Autodesk Inventor part; units mm, degrees
(part 2 of 3)
  line L469 (15.7875, 18.7015) -> (16.0329, 18.7015) construction
  spline S155 degree 3 poles (16.0329, 18.7015) (16.2784, 18.7015) (16.4775, 18.9006) (16.4775, 19.1461) knots 0 0 0 0 1 1 1 1
  line L470 (16.0329, 18.7015) -> (16.2784, 18.7015) construction
  line L471 (16.2784, 18.7015) -> (16.4775, 18.9006) construction
  line L472 (16.4775, 18.9006) -> (16.4775, 19.1461) construction
  spline S156 degree 3 poles (11.3975, 19.1461) (11.3975, 19.3915) (11.1984, 19.5905) (10.9529, 19.5905) knots 0 0 0 0 1 1 1 1
  line L473 (11.3975, 19.1461) -> (11.3975, 19.3915) construction
  line L474 (11.3975, 19.3915) -> (11.1984, 19.5905) construction
  line L475 (11.1984, 19.5905) -> (10.9529, 19.5905) construction
  spline S157 degree 3 poles (10.9529, 19.5905) (10.7075, 19.5905) (10.5085, 19.3915) (10.5085, 19.1461) knots 0 0 0 0 1 1 1 1
  line L476 (10.9529, 19.5905) -> (10.7075, 19.5905) construction
  line L477 (10.7075, 19.5905) -> (10.5085, 19.3915) construction
  line L478 (10.5085, 19.3915) -> (10.5085, 19.1461) construction
  spline S158 degree 3 poles (10.5085, 19.1461) (10.5085, 18.9006) (10.7075, 18.7015) (10.9529, 18.7015) knots 0 0 0 0 1 1 1 1
  line L479 (10.5085, 19.1461) -> (10.5085, 18.9006) construction
  line L480 (10.5085, 18.9006) -> (10.7075, 18.7015) construction
  line L481 (10.7075, 18.7015) -> (10.9529, 18.7015) construction
  spline S159 degree 3 poles (10.9529, 18.7015) (11.1984, 18.7015) (11.3975, 18.9006) (11.3975, 19.1461) knots 0 0 0 0 1 1 1 1
  line L482 (10.9529, 18.7015) -> (11.1984, 18.7015) construction
  line L483 (11.1984, 18.7015) -> (11.3975, 18.9006) construction
  line L484 (11.3975, 18.9006) -> (11.3975, 19.1461) construction
  spline S160 degree 3 poles (8.8575, 19.1461) (8.8575, 19.3915) (8.6584, 19.5905) (8.4129, 19.5905) knots 0 0 0 0 1 1 1 1
  line L485 (8.8575, 19.1461) -> (8.8575, 19.3915) construction
  line L486 (8.8575, 19.3915) -> (8.6584, 19.5905) construction
  line L487 (8.6584, 19.5905) -> (8.4129, 19.5905) construction
  spline S161 degree 3 poles (8.4129, 19.5905) (8.1675, 19.5905) (7.9685, 19.3915) (7.9685, 19.1461) knots 0 0 0 0 1 1 1 1
  line L488 (8.4129, 19.5905) -> (8.1675, 19.5905) construction
  line L489 (8.1675, 19.5905) -> (7.9685, 19.3915) construction
  line L490 (7.9685, 19.3915) -> (7.9685, 19.1461) construction
  spline S162 degree 3 poles (7.9685, 19.1461) (7.9685, 18.9006) (8.1675, 18.7015) (8.4129, 18.7015) knots 0 0 0 0 1 1 1 1
  line L491 (7.9685, 19.1461) -> (7.9685, 18.9006) construction
  line L492 (7.9685, 18.9006) -> (8.1675, 18.7015) construction
  line L493 (8.1675, 18.7015) -> (8.4129, 18.7015) construction
  spline S163 degree 3 poles (8.4129, 18.7015) (8.6584, 18.7015) (8.8575, 18.9006) (8.8575, 19.1461) knots 0 0 0 0 1 1 1 1
  line L494 (8.4129, 18.7015) -> (8.6584, 18.7015) construction
  line L495 (8.6584, 18.7015) -> (8.8575, 18.9006) construction
  line L496 (8.8575, 18.9006) -> (8.8575, 19.1461) construction
  spline S164 degree 3 poles (6.3175, 19.1461) (6.3175, 19.3915) (6.1184, 19.5905) (5.8729, 19.5905) knots 0 0 0 0 1 1 1 1
  line L497 (6.3175, 19.1461) -> (6.3175, 19.3915) construction
  line L498 (6.3175, 19.3915) -> (6.1184, 19.5905) construction
  line L499 (6.1184, 19.5905) -> (5.8729, 19.5905) construction
  spline S165 degree 3 poles (5.8729, 19.5905) (5.6275, 19.5905) (5.4285, 19.3915) (5.4285, 19.1461) knots 0 0 0 0 1 1 1 1
  line L500 (5.8729, 19.5905) -> (5.6275, 19.5905) construction
  line L501 (5.6275, 19.5905) -> (5.4285, 19.3915) construction
  line L502 (5.4285, 19.3915) -> (5.4285, 19.1461) construction
  spline S166 degree 3 poles (5.4285, 19.1461) (5.4285, 18.9006) (5.6275, 18.7015) (5.8729, 18.7015) knots 0 0 0 0 1 1 1 1
  line L503 (5.4285, 19.1461) -> (5.4285, 18.9006) construction
  line L504 (5.4285, 18.9006) -> (5.6275, 18.7015) construction
  line L505 (5.6275, 18.7015) -> (5.8729, 18.7015) construction
  spline S167 degree 3 poles (5.8729, 18.7015) (6.1184, 18.7015) (6.3175, 18.9006) (6.3175, 19.1461) knots 0 0 0 0 1 1 1 1
  line L506 (5.8729, 18.7015) -> (6.1184, 18.7015) construction
  line L507 (6.1184, 18.7015) -> (6.3175, 18.9006) construction
  line L508 (6.3175, 18.9006) -> (6.3175, 19.1461) construction
  spline S168 degree 3 poles (6.3175, 15.3361) (6.3175, 15.5815) (6.1184, 15.7805) (5.8729, 15.7805) knots 0 0 0 0 1 1 1 1
  line L509 (6.3175, 15.3361) -> (6.3175, 15.5815) construction
  line L510 (6.3175, 15.5815) -> (6.1184, 15.7805) construction
  line L511 (6.1184, 15.7805) -> (5.8729, 15.7805) construction
  spline S169 degree 3 poles (5.8729, 15.7805) (5.6275, 15.7805) (5.4285, 15.5815) (5.4285, 15.3361) knots 0 0 0 0 1 1 1 1
  line L512 (5.8729, 15.7805) -> (5.6275, 15.7805) construction
  line L513 (5.6275, 15.7805) -> (5.4285, 15.5815) construction
  line L514 (5.4285, 15.5815) -> (5.4285, 15.3361) construction
  spline S170 degree 3 poles (5.4285, 15.3361) (5.4285, 15.0906) (5.6275, 14.8915) (5.8729, 14.8915) knots 0 0 0 0 1 1 1 1
  line L515 (5.4285, 15.3361) -> (5.4285, 15.0906) construction
  line L516 (5.4285, 15.0906) -> (5.6275, 14.8915) construction
  line L517 (5.6275, 14.8915) -> (5.8729, 14.8915) construction
  spline S171 degree 3 poles (5.8729, 14.8915) (6.1184, 14.8915) (6.3175, 15.0906) (6.3175, 15.3361) knots 0 0 0 0 1 1 1 1
  line L518 (5.8729, 14.8915) -> (6.1184, 14.8915) construction
  line L519 (6.1184, 14.8915) -> (6.3175, 15.0906) construction
  line L520 (6.3175, 15.0906) -> (6.3175, 15.3361) construction
  spline S172 degree 3 poles (8.8575, 15.3361) (8.8575, 15.5815) (8.6584, 15.7805) (8.4129, 15.7805) knots 0 0 0 0 1 1 1 1
  line L521 (8.8575, 15.3361) -> (8.8575, 15.5815) construction
  line L522 (8.8575, 15.5815) -> (8.6584, 15.7805) construction
  line L523 (8.6584, 15.7805) -> (8.4129, 15.7805) construction
  spline S173 degree 3 poles (8.4129, 15.7805) (8.1675, 15.7805) (7.9685, 15.5815) (7.9685, 15.3361) knots 0 0 0 0 1 1 1 1
  line L524 (8.4129, 15.7805) -> (8.1675, 15.7805) construction
  line L525 (8.1675, 15.7805) -> (7.9685, 15.5815) construction
  line L526 (7.9685, 15.5815) -> (7.9685, 15.3361) construction
  spline S174 degree 3 poles (7.9685, 15.3361) (7.9685, 15.0906) (8.1675, 14.8915) (8.4129, 14.8915) knots 0 0 0 0 1 1 1 1
  line L527 (7.9685, 15.3361) -> (7.9685, 15.0906) construction
  line L528 (7.9685, 15.0906) -> (8.1675, 14.8915) construction
  line L529 (8.1675, 14.8915) -> (8.4129, 14.8915) construction
  spline S175 degree 3 poles (8.4129, 14.8915) (8.6584, 14.8915) (8.8575, 15.0906) (8.8575, 15.3361) knots 0 0 0 0 1 1 1 1
  line L530 (8.4129, 14.8915) -> (8.6584, 14.8915) construction
  line L531 (8.6584, 14.8915) -> (8.8575, 15.0906) construction
  line L532 (8.8575, 15.0906) -> (8.8575, 15.3361) construction
  spline S176 degree 3 poles (19.0175, 19.1461) (19.0175, 19.3915) (18.8184, 19.5905) (18.5729, 19.5905) knots 0 0 0 0 1 1 1 1
  line L533 (19.0175, 19.1461) -> (19.0175, 19.3915) construction
  line L534 (19.0175, 19.3915) -> (18.8184, 19.5905) construction
  line L535 (18.8184, 19.5905) -> (18.5729, 19.5905) construction
  spline S177 degree 3 poles (18.5729, 19.5905) (18.3275, 19.5905) (18.1285, 19.3915) (18.1285, 19.1461) knots 0 0 0 0 1 1 1 1
  line L536 (18.5729, 19.5905) -> (18.3275, 19.5905) construction
  line L537 (18.3275, 19.5905) -> (18.1285, 19.3915) construction
  line L538 (18.1285, 19.3915) -> (18.1285, 19.1461) construction
  spline S178 degree 3 poles (18.1285, 19.1461) (18.1285, 18.9006) (18.3275, 18.7015) (18.5729, 18.7015) knots 0 0 0 0 1 1 1 1
  line L539 (18.1285, 19.1461) -> (18.1285, 18.9006) construction
  line L540 (18.1285, 18.9006) -> (18.3275, 18.7015) construction
  line L541 (18.3275, 18.7015) -> (18.5729, 18.7015) construction
  spline S179 degree 3 poles (18.5729, 18.7015) (18.8184, 18.7015) (19.0175, 18.9006) (19.0175, 19.1461) knots 0 0 0 0 1 1 1 1
  line L542 (18.5729, 18.7015) -> (18.8184, 18.7015) construction
  line L543 (18.8184, 18.7015) -> (19.0175, 18.9006) construction
  line L544 (19.0175, 18.9006) -> (19.0175, 19.1461) construction
  spline S180 degree 3 poles (21.5575, 19.1461) (21.5575, 19.3915) (21.3584, 19.5905) (21.1129, 19.5905) knots 0 0 0 0 1 1 1 1
  line L545 (21.5575, 19.1461) -> (21.5575, 19.3915) construction
  line L546 (21.5575, 19.3915) -> (21.3584, 19.5905) construction
  line L547 (21.3584, 19.5905) -> (21.1129, 19.5905) construction
  spline S181 degree 3 poles (21.1129, 19.5905) (20.8675, 19.5905) (20.6685, 19.3915) (20.6685, 19.1461) knots 0 0 0 0 1 1 1 1
  line L548 (21.1129, 19.5905) -> (20.8675, 19.5905) construction
  line L549 (20.8675, 19.5905) -> (20.6685, 19.3915) construction
  line L550 (20.6685, 19.3915) -> (20.6685, 19.1461) construction
  spline S182 degree 3 poles (20.6685, 19.1461) (20.6685, 18.9006) (20.8675, 18.7015) (21.1129, 18.7015) knots 0 0 0 0 1 1 1 1
  line L551 (20.6685, 19.1461) -> (20.6685, 18.9006) construction
  line L552 (20.6685, 18.9006) -> (20.8675, 18.7015) construction
  line L553 (20.8675, 18.7015) -> (21.1129, 18.7015) construction
  spline S183 degree 3 poles (21.1129, 18.7015) (21.3584, 18.7015) (21.5575, 18.9006) (21.5575, 19.1461) knots 0 0 0 0 1 1 1 1
  line L554 (21.1129, 18.7015) -> (21.3584, 18.7015) construction
  line L555 (21.3584, 18.7015) -> (21.5575, 18.9006) construction
  line L556 (21.5575, 18.9006) -> (21.5575, 19.1461) construction
  spline S184 degree 3 poles (24.0975, 19.1461) (24.0975, 19.3915) (23.8984, 19.5905) (23.6529, 19.5905) knots 0 0 0 0 1 1 1 1
  line L557 (24.0975, 19.1461) -> (24.0975, 19.3915) construction
  line L558 (24.0975, 19.3915) -> (23.8984, 19.5905) construction
  line L559 (23.8984, 19.5905) -> (23.6529, 19.5905) construction
  spline S185 degree 3 poles (23.6529, 19.5905) (23.4075, 19.5905) (23.2085, 19.3915) (23.2085, 19.1461) knots 0 0 0 0 1 1 1 1
  line L560 (23.6529, 19.5905) -> (23.4075, 19.5905) construction
  line L561 (23.4075, 19.5905) -> (23.2085, 19.3915) construction
  line L562 (23.2085, 19.3915) -> (23.2085, 19.1461) construction
  spline S186 degree 3 poles (23.2085, 19.1461) (23.2085, 18.9006) (23.4075, 18.7015) (23.6529, 18.7015) knots 0 0 0 0 1 1 1 1
  line L563 (23.2085, 19.1461) -> (23.2085, 18.9006) construction
  line L564 (23.2085, 18.9006) -> (23.4075, 18.7015) construction
  line L565 (23.4075, 18.7015) -> (23.6529, 18.7015) construction
  spline S187 degree 3 poles (23.6529, 18.7015) (23.8984, 18.7015) (24.0975, 18.9006) (24.0975, 19.1461) knots 0 0 0 0 1 1 1 1
  line L566 (23.6529, 18.7015) -> (23.8984, 18.7015) construction
  line L567 (23.8984, 18.7015) -> (24.0975, 18.9006) construction
  line L568 (24.0975, 18.9006) -> (24.0975, 19.1461) construction
  spline S188 degree 3 poles (11.3975, 15.3361) (11.3975, 15.5815) (11.1984, 15.7805) (10.9529, 15.7805) knots 0 0 0 0 1 1 1 1
  line L569 (11.3975, 15.3361) -> (11.3975, 15.5815) construction
  line L570 (11.3975, 15.5815) -> (11.1984, 15.7805) construction
  line L571 (11.1984, 15.7805) -> (10.9529, 15.7805) construction
  spline S189 degree 3 poles (10.9529, 15.7805) (10.7075, 15.7805) (10.5085, 15.5815) (10.5085, 15.3361) knots 0 0 0 0 1 1 1 1
  line L572 (10.9529, 15.7805) -> (10.7075, 15.7805) construction
  line L573 (10.7075, 15.7805) -> (10.5085, 15.5815) construction
  line L574 (10.5085, 15.5815) -> (10.5085, 15.3361) construction
  spline S190 degree 3 poles (10.5085, 15.3361) (10.5085, 15.0906) (10.7075, 14.8915) (10.9529, 14.8915) knots 0 0 0 0 1 1 1 1
  line L575 (10.5085, 15.3361) -> (10.5085, 15.0906) construction
  line L576 (10.5085, 15.0906) -> (10.7075, 14.8915) construction
  line L577 (10.7075, 14.8915) -> (10.9529, 14.8915) construction
  spline S191 degree 3 poles (10.9529, 14.8915) (11.1984, 14.8915) (11.3975, 15.0906) (11.3975, 15.3361) knots 0 0 0 0 1 1 1 1
  line L578 (10.9529, 14.8915) -> (11.1984, 14.8915) construction
  line L579 (11.1984, 14.8915) -> (11.3975, 15.0906) construction
  line L580 (11.3975, 15.0906) -> (11.3975, 15.3361) construction
  spline S192 degree 3 poles (13.9375, 15.3361) (13.9375, 15.5815) (13.7384, 15.7805) (13.4929, 15.7805) knots 0 0 0 0 1 1 1 1
  line L581 (13.9375, 15.3361) -> (13.9375, 15.5815) construction
  line L582 (13.9375, 15.5815) -> (13.7384, 15.7805) construction
  line L583 (13.7384, 15.7805) -> (13.4929, 15.7805) construction
  spline S193 degree 3 poles (13.4929, 15.7805) (13.2475, 15.7805) (13.0485, 15.5815) (13.0485, 15.3361) knots 0 0 0 0 1 1 1 1
  line L584 (13.4929, 15.7805) -> (13.2475, 15.7805) construction
  line L585 (13.2475, 15.7805) -> (13.0485, 15.5815) construction
  line L586 (13.0485, 15.5815) -> (13.0485, 15.3361) construction
  spline S194 degree 3 poles (13.0485, 15.3361) (13.0485, 15.0906) (13.2475, 14.8915) (13.4929, 14.8915) knots 0 0 0 0 1 1 1 1
  line L587 (13.0485, 15.3361) -> (13.0485, 15.0906) construction
  line L588 (13.0485, 15.0906) -> (13.2475, 14.8915) construction
  line L589 (13.2475, 14.8915) -> (13.4929, 14.8915) construction
  spline S195 degree 3 poles (13.4929, 14.8915) (13.7384, 14.8915) (13.9375, 15.0906) (13.9375, 15.3361) knots 0 0 0 0 1 1 1 1
  line L590 (13.4929, 14.8915) -> (13.7384, 14.8915) construction
  line L591 (13.7384, 14.8915) -> (13.9375, 15.0906) construction
  line L592 (13.9375, 15.0906) -> (13.9375, 15.3361) construction
  spline S196 degree 3 poles (16.4775, 15.3361) (16.4775, 15.5815) (16.2784, 15.7805) (16.0329, 15.7805) knots 0 0 0 0 1 1 1 1
  line L593 (16.4775, 15.3361) -> (16.4775, 15.5815) construction
  line L594 (16.4775, 15.5815) -> (16.2784, 15.7805) construction
  line L595 (16.2784, 15.7805) -> (16.0329, 15.7805) construction
  spline S197 degree 3 poles (16.0329, 15.7805) (15.7875, 15.7805) (15.5885, 15.5815) (15.5885, 15.3361) knots 0 0 0 0 1 1 1 1
  line L596 (16.0329, 15.7805) -> (15.7875, 15.7805) construction
  line L597 (15.7875, 15.7805) -> (15.5885, 15.5815) construction
  line L598 (15.5885, 15.5815) -> (15.5885, 15.3361) construction
  spline S198 degree 3 poles (15.5885, 15.3361) (15.5885, 15.0906) (15.7875, 14.8915) (16.0329, 14.8915) knots 0 0 0 0 1 1 1 1
  line L599 (15.5885, 15.3361) -> (15.5885, 15.0906) construction
  line L600 (15.5885, 15.0906) -> (15.7875, 14.8915) construction
  line L601 (15.7875, 14.8915) -> (16.0329, 14.8915) construction
  spline S199 degree 3 poles (16.0329, 14.8915) (16.2784, 14.8915) (16.4775, 15.0906) (16.4775, 15.3361) knots 0 0 0 0 1 1 1 1
  line L602 (16.0329, 14.8915) -> (16.2784, 14.8915) construction
  line L603 (16.2784, 14.8915) -> (16.4775, 15.0906) construction
  line L604 (16.4775, 15.0906) -> (16.4775, 15.3361) construction
  spline S200 degree 3 poles (19.0175, 15.3361) (19.0175, 15.5815) (18.8184, 15.7805) (18.5729, 15.7805) knots 0 0 0 0 1 1 1 1
  line L605 (19.0175, 15.3361) -> (19.0175, 15.5815) construction
  line L606 (19.0175, 15.5815) -> (18.8184, 15.7805) construction
  line L607 (18.8184, 15.7805) -> (18.5729, 15.7805) construction
  spline S201 degree 3 poles (18.5729, 15.7805) (18.3275, 15.7805) (18.1285, 15.5815) (18.1285, 15.3361) knots 0 0 0 0 1 1 1 1
  line L608 (18.5729, 15.7805) -> (18.3275, 15.7805) construction
  line L609 (18.3275, 15.7805) -> (18.1285, 15.5815) construction
  line L610 (18.1285, 15.5815) -> (18.1285, 15.3361) construction
  spline S202 degree 3 poles (18.1285, 15.3361) (18.1285, 15.0906) (18.3275, 14.8915) (18.5729, 14.8915) knots 0 0 0 0 1 1 1 1
  line L611 (18.1285, 15.3361) -> (18.1285, 15.0906) construction
  line L612 (18.1285, 15.0906) -> (18.3275, 14.8915) construction
  line L613 (18.3275, 14.8915) -> (18.5729, 14.8915) construction
  spline S203 degree 3 poles (18.5729, 14.8915) (18.8184, 14.8915) (19.0175, 15.0906) (19.0175, 15.3361) knots 0 0 0 0 1 1 1 1
  line L614 (18.5729, 14.8915) -> (18.8184, 14.8915) construction
  line L615 (18.8184, 14.8915) -> (19.0175, 15.0906) construction
  line L616 (19.0175, 15.0906) -> (19.0175, 15.3361) construction
  spline S204 degree 3 poles (21.5575, 15.3361) (21.5575, 15.5815) (21.3584, 15.7805) (21.1129, 15.7805) knots 0 0 0 0 1 1 1 1
  line L617 (21.5575, 15.3361) -> (21.5575, 15.5815) construction
  line L618 (21.5575, 15.5815) -> (21.3584, 15.7805) construction
  line L619 (21.3584, 15.7805) -> (21.1129, 15.7805) construction
  spline S205 degree 3 poles (21.1129, 15.7805) (20.8675, 15.7805) (20.6685, 15.5815) (20.6685, 15.3361) knots 0 0 0 0 1 1 1 1
  line L620 (21.1129, 15.7805) -> (20.8675, 15.7805) construction
  line L621 (20.8675, 15.7805) -> (20.6685, 15.5815) construction
  line L622 (20.6685, 15.5815) -> (20.6685, 15.3361) construction
  spline S206 degree 3 poles (20.6685, 15.3361) (20.6685, 15.0906) (20.8675, 14.8915) (21.1129, 14.8915) knots 0 0 0 0 1 1 1 1
  line L623 (20.6685, 15.3361) -> (20.6685, 15.0906) construction
  line L624 (20.6685, 15.0906) -> (20.8675, 14.8915) construction
  line L625 (20.8675, 14.8915) -> (21.1129, 14.8915) construction
  spline S207 degree 3 poles (21.1129, 14.8915) (21.3584, 14.8915) (21.5575, 15.0906) (21.5575, 15.3361) knots 0 0 0 0 1 1 1 1
  line L626 (21.1129, 14.8915) -> (21.3584, 14.8915) construction
  line L627 (21.3584, 14.8915) -> (21.5575, 15.0906) construction
  line L628 (21.5575, 15.0906) -> (21.5575, 15.3361) construction
  spline S208 degree 3 poles (24.0975, 15.3361) (24.0975, 15.5815) (23.8984, 15.7805) (23.6529, 15.7805) knots 0 0 0 0 1 1 1 1
  line L629 (24.0975, 15.3361) -> (24.0975, 15.5815) construction
  line L630 (24.0975, 15.5815) -> (23.8984, 15.7805) construction
  line L631 (23.8984, 15.7805) -> (23.6529, 15.7805) construction
  spline S209 degree 3 poles (23.6529, 15.7805) (23.4075, 15.7805) (23.2085, 15.5815) (23.2085, 15.3361) knots 0 0 0 0 1 1 1 1
  line L632 (23.6529, 15.7805) -> (23.4075, 15.7805) construction
  line L633 (23.4075, 15.7805) -> (23.2085, 15.5815) construction
  line L634 (23.2085, 15.5815) -> (23.2085, 15.3361) construction
  spline S210 degree 3 poles (23.2085, 15.3361) (23.2085, 15.0906) (23.4075, 14.8915) (23.6529, 14.8915) knots 0 0 0 0 1 1 1 1
  line L635 (23.2085, 15.3361) -> (23.2085, 15.0906) construction
  line L636 (23.2085, 15.0906) -> (23.4075, 14.8915) construction
  line L637 (23.4075, 14.8915) -> (23.6529, 14.8915) construction
  spline S211 degree 3 poles (23.6529, 14.8915) (23.8984, 14.8915) (24.0975, 15.0906) (24.0975, 15.3361) knots 0 0 0 0 1 1 1 1
  line L638 (23.6529, 14.8915) -> (23.8984, 14.8915) construction
  line L639 (23.8984, 14.8915) -> (24.0975, 15.0906) construction
  line L640 (24.0975, 15.0906) -> (24.0975, 15.3361) construction
  spline S212 degree 3 poles (13.9375, 29.3061) (13.9375, 29.5515) (13.7384, 29.7505) (13.4929, 29.7505) knots 0 0 0 0 1 1 1 1
  line L641 (13.9375, 29.3061) -> (13.9375, 29.5515) construction
  line L642 (13.9375, 29.5515) -> (13.7384, 29.7505) construction
  line L643 (13.7384, 29.7505) -> (13.4929, 29.7505) construction
  spline S213 degree 3 poles (13.4929, 29.7505) (13.2475, 29.7505) (13.0485, 29.5515) (13.0485, 29.3061) knots 0 0 0 0 1 1 1 1
  line L644 (13.4929, 29.7505) -> (13.2475, 29.7505) construction
  line L645 (13.2475, 29.7505) -> (13.0485, 29.5515) construction
  line L646 (13.0485, 29.5515) -> (13.0485, 29.3061) construction
  spline S214 degree 3 poles (13.0485, 29.3061) (13.0485, 29.0606) (13.2475, 28.8615) (13.4929, 28.8615) knots 0 0 0 0 1 1 1 1
  line L647 (13.0485, 29.3061) -> (13.0485, 29.0606) construction
  line L648 (13.0485, 29.0606) -> (13.2475, 28.8615) construction
  line L649 (13.2475, 28.8615) -> (13.4929, 28.8615) construction
  spline S215 degree 3 poles (13.4929, 28.8615) (13.7384, 28.8615) (13.9375, 29.0606) (13.9375, 29.3061) knots 0 0 0 0 1 1 1 1
  line L650 (13.4929, 28.8615) -> (13.7384, 28.8615) construction
  line L651 (13.7384, 28.8615) -> (13.9375, 29.0606) construction
  line L652 (13.9375, 29.0606) -> (13.9375, 29.3061) construction
  spline S216 degree 3 poles (16.4775, 29.3061) (16.4775, 29.5515) (16.2784, 29.7505) (16.0329, 29.7505) knots 0 0 0 0 1 1 1 1
  line L653 (16.4775, 29.3061) -> (16.4775, 29.5515) construction
  line L654 (16.4775, 29.5515) -> (16.2784, 29.7505) construction
  line L655 (16.2784, 29.7505) -> (16.0329, 29.7505) construction
  spline S217 degree 3 poles (16.0329, 29.7505) (15.7875, 29.7505) (15.5885, 29.5515) (15.5885, 29.3061) knots 0 0 0 0 1 1 1 1
  line L656 (16.0329, 29.7505) -> (15.7875, 29.7505) construction
  line L657 (15.7875, 29.7505) -> (15.5885, 29.5515) construction
  line L658 (15.5885, 29.5515) -> (15.5885, 29.3061) construction
  spline S218 degree 3 poles (15.5885, 29.3061) (15.5885, 29.0606) (15.7875, 28.8615) (16.0329, 28.8615) knots 0 0 0 0 1 1 1 1
  line L659 (15.5885, 29.3061) -> (15.5885, 29.0606) construction
  line L660 (15.5885, 29.0606) -> (15.7875, 28.8615) construction
  line L661 (15.7875, 28.8615) -> (16.0329, 28.8615) construction
  spline S219 degree 3 poles (16.0329, 28.8615) (16.2784, 28.8615) (16.4775, 29.0606) (16.4775, 29.3061) knots 0 0 0 0 1 1 1 1
  line L662 (16.0329, 28.8615) -> (16.2784, 28.8615) construction
  line L663 (16.2784, 28.8615) -> (16.4775, 29.0606) construction
  line L664 (16.4775, 29.0606) -> (16.4775, 29.3061) construction
  spline S220 degree 3 poles (11.3975, 29.3061) (11.3975, 29.5515) (11.1984, 29.7505) (10.9529, 29.7505) knots 0 0 0 0 1 1 1 1
  line L665 (11.3975, 29.3061) -> (11.3975, 29.5515) construction
  line L666 (11.3975, 29.5515) -> (11.1984, 29.7505) construction
  line L667 (11.1984, 29.7505) -> (10.9529, 29.7505) construction
  spline S221 degree 3 poles (10.9529, 29.7505) (10.7075, 29.7505) (10.5085, 29.5515) (10.5085, 29.3061) knots 0 0 0 0 1 1 1 1
  line L668 (10.9529, 29.7505) -> (10.7075, 29.7505) construction
  line L669 (10.7075, 29.7505) -> (10.5085, 29.5515) construction
  line L670 (10.5085, 29.5515) -> (10.5085, 29.3061) construction
  spline S222 degree 3 poles (10.5085, 29.3061) (10.5085, 29.0606) (10.7075, 28.8615) (10.9529, 28.8615) knots 0 0 0 0 1 1 1 1
  line L671 (10.5085, 29.3061) -> (10.5085, 29.0606) construction
  line L672 (10.5085, 29.0606) -> (10.7075, 28.8615) construction
  line L673 (10.7075, 28.8615) -> (10.9529, 28.8615) construction
  spline S223 degree 3 poles (10.9529, 28.8615) (11.1984, 28.8615) (11.3975, 29.0606) (11.3975, 29.3061) knots 0 0 0 0 1 1 1 1
  line L674 (10.9529, 28.8615) -> (11.1984, 28.8615) construction
  line L675 (11.1984, 28.8615) -> (11.3975, 29.0606) construction
  line L676 (11.3975, 29.0606) -> (11.3975, 29.3061) construction
  spline S224 degree 3 poles (19.0175, 29.3061) (19.0175, 29.5515) (18.8184, 29.7505) (18.5729, 29.7505) knots 0 0 0 0 1 1 1 1
  line L677 (19.0175, 29.3061) -> (19.0175, 29.5515) construction
  line L678 (19.0175, 29.5515) -> (18.8184, 29.7505) construction
  line L679 (18.8184, 29.7505) -> (18.5729, 29.7505) construction
  spline S225 degree 3 poles (18.5729, 29.7505) (18.3275, 29.7505) (18.1285, 29.5515) (18.1285, 29.3061) knots 0 0 0 0 1 1 1 1
  line L680 (18.5729, 29.7505) -> (18.3275, 29.7505) construction
  line L681 (18.3275, 29.7505) -> (18.1285, 29.5515) construction
  line L682 (18.1285, 29.5515) -> (18.1285, 29.3061) construction
  spline S226 degree 3 poles (18.1285, 29.3061) (18.1285, 29.0606) (18.3275, 28.8615) (18.5729, 28.8615) knots 0 0 0 0 1 1 1 1
  line L683 (18.1285, 29.3061) -> (18.1285, 29.0606) construction
  line L684 (18.1285, 29.0606) -> (18.3275, 28.8615) construction
  line L685 (18.3275, 28.8615) -> (18.5729, 28.8615) construction
  spline S227 degree 3 poles (18.5729, 28.8615) (18.8184, 28.8615) (19.0175, 29.0606) (19.0175, 29.3061) knots 0 0 0 0 1 1 1 1
  line L686 (18.5729, 28.8615) -> (18.8184, 28.8615) construction
  line L687 (18.8184, 28.8615) -> (19.0175, 29.0606) construction
  line L688 (19.0175, 29.0606) -> (19.0175, 29.3061) construction
  spline S228 degree 3 poles (21.5575, 29.3061) (21.5575, 29.5515) (21.3584, 29.7505) (21.1129, 29.7505) knots 0 0 0 0 1 1 1 1
  line L689 (21.5575, 29.3061) -> (21.5575, 29.5515) construction
  line L690 (21.5575, 29.5515) -> (21.3584, 29.7505) construction
  line L691 (21.3584, 29.7505) -> (21.1129, 29.7505) construction
  spline S229 degree 3 poles (21.1129, 29.7505) (20.8675, 29.7505) (20.6685, 29.5515) (20.6685, 29.3061) knots 0 0 0 0 1 1 1 1
  line L692 (21.1129, 29.7505) -> (20.8675, 29.7505) construction
  line L693 (20.8675, 29.7505) -> (20.6685, 29.5515) construction
  line L694 (20.6685, 29.5515) -> (20.6685, 29.3061) construction
  spline S230 degree 3 poles (20.6685, 29.3061) (20.6685, 29.0606) (20.8675, 28.8615) (21.1129, 28.8615) knots 0 0 0 0 1 1 1 1
  line L695 (20.6685, 29.3061) -> (20.6685, 29.0606) construction
  line L696 (20.6685, 29.0606) -> (20.8675, 28.8615) construction
  line L697 (20.8675, 28.8615) -> (21.1129, 28.8615) construction
  spline S231 degree 3 poles (21.1129, 28.8615) (21.3584, 28.8615) (21.5575, 29.0606) (21.5575, 29.3061) knots 0 0 0 0 1 1 1 1
  line L698 (21.1129, 28.8615) -> (21.3584, 28.8615) construction
  line L699 (21.3584, 28.8615) -> (21.5575, 29.0606) construction
  line L700 (21.5575, 29.0606) -> (21.5575, 29.3061) construction
  spline S232 degree 3 poles (24.0975, 29.3061) (24.0975, 29.5515) (23.8984, 29.7505) (23.6529, 29.7505) knots 0 0 0 0 1 1 1 1
  line L701 (24.0975, 29.3061) -> (24.0975, 29.5515) construction
  line L702 (24.0975, 29.5515) -> (23.8984, 29.7505) construction
  line L703 (23.8984, 29.7505) -> (23.6529, 29.7505) construction
  spline S233 degree 3 poles (23.6529, 29.7505) (23.4075, 29.7505) (23.2085, 29.5515) (23.2085, 29.3061) knots 0 0 0 0 1 1 1 1
  line L704 (23.6529, 29.7505) -> (23.4075, 29.7505) construction
  line L705 (23.4075, 29.7505) -> (23.2085, 29.5515) construction
  line L706 (23.2085, 29.5515) -> (23.2085, 29.3061) construction
  spline S234 degree 3 poles (23.2085, 29.3061) (23.2085, 29.0606) (23.4075, 28.8615) (23.6529, 28.8615) knots 0 0 0 0 1 1 1 1
  line L707 (23.2085, 29.3061) -> (23.2085, 29.0606) construction
  line L708 (23.2085, 29.0606) -> (23.4075, 28.8615) construction
  line L709 (23.4075, 28.8615) -> (23.6529, 28.8615) construction
  spline S235 degree 3 poles (23.6529, 28.8615) (23.8984, 28.8615) (24.0975, 29.0606) (24.0975, 29.3061) knots 0 0 0 0 1 1 1 1
  line L710 (23.6529, 28.8615) -> (23.8984, 28.8615) construction
  line L711 (23.8984, 28.8615) -> (24.0975, 29.0606) construction
  line L712 (24.0975, 29.0606) -> (24.0975, 29.3061) construction
  spline S236 degree 3 poles (8.8575, 29.3061) (8.8575, 29.5515) (8.6584, 29.7505) (8.4129, 29.7505) knots 0 0 0 0 1 1 1 1
  line L713 (8.8575, 29.3061) -> (8.8575, 29.5515) construction
  line L714 (8.8575, 29.5515) -> (8.6584, 29.7505) construction
  line L715 (8.6584, 29.7505) -> (8.4129, 29.7505) construction
  spline S237 degree 3 poles (8.4129, 29.7505) (8.1675, 29.7505) (7.9685, 29.5515) (7.9685, 29.3061) knots 0 0 0 0 1 1 1 1
  line L716 (8.4129, 29.7505) -> (8.1675, 29.7505) construction
  line L717 (8.1675, 29.7505) -> (7.9685, 29.5515) construction
  line L718 (7.9685, 29.5515) -> (7.9685, 29.3061) construction
  spline S238 degree 3 poles (7.9685, 29.3061) (7.9685, 29.0606) (8.1675, 28.8615) (8.4129, 28.8615) knots 0 0 0 0 1 1 1 1
  line L719 (7.9685, 29.3061) -> (7.9685, 29.0606) construction
  line L720 (7.9685, 29.0606) -> (8.1675, 28.8615) construction
  line L721 (8.1675, 28.8615) -> (8.4129, 28.8615) construction
  spline S239 degree 3 poles (8.4129, 28.8615) (8.6584, 28.8615) (8.8575, 29.0606) (8.8575, 29.3061) knots 0 0 0 0 1 1 1 1
  line L722 (8.4129, 28.8615) -> (8.6584, 28.8615) construction
  line L723 (8.6584, 28.8615) -> (8.8575, 29.0606) construction
  line L724 (8.8575, 29.0606) -> (8.8575, 29.3061) construction
  spline S240 degree 3 poles (6.3175, 29.3061) (6.3175, 29.5515) (6.1184, 29.7505) (5.8729, 29.7505) knots 0 0 0 0 1 1 1 1
  line L725 (6.3175, 29.3061) -> (6.3175, 29.5515) construction
  line L726 (6.3175, 29.5515) -> (6.1184, 29.7505) construction
  line L727 (6.1184, 29.7505) -> (5.8729, 29.7505) construction
  spline S241 degree 3 poles (5.8729, 29.7505) (5.6275, 29.7505) (5.4285, 29.5515) (5.4285, 29.3061) knots 0 0 0 0 1 1 1 1
  line L728 (5.8729, 29.7505) -> (5.6275, 29.7505) construction
  line L729 (5.6275, 29.7505) -> (5.4285, 29.5515) construction
  line L730 (5.4285, 29.5515) -> (5.4285, 29.3061) construction
  spline S242 degree 3 poles (5.4285, 29.3061) (5.4285, 29.0606) (5.6275, 28.8615) (5.8729, 28.8615) knots 0 0 0 0 1 1 1 1
  line L731 (5.4285, 29.3061) -> (5.4285, 29.0606) construction
  line L732 (5.4285, 29.0606) -> (5.6275, 28.8615) construction
  line L733 (5.6275, 28.8615) -> (5.8729, 28.8615) construction
  spline S243 degree 3 poles (5.8729, 28.8615) (6.1184, 28.8615) (6.3175, 29.0606) (6.3175, 29.3061) knots 0 0 0 0 1 1 1 1
  line L734 (5.8729, 28.8615) -> (6.1184, 28.8615) construction
  line L735 (6.1184, 28.8615) -> (6.3175, 29.0606) construction
  line L736 (6.3175, 29.0606) -> (6.3175, 29.3061) construction
  spline S244 degree 3 poles (6.3175, 33.1161) (6.3175, 33.3615) (6.1184, 33.5605) (5.8729, 33.5605) knots 0 0 0 0 1 1 1 1
  line L737 (6.3175, 33.1161) -> (6.3175, 33.3615) construction
  line L738 (6.3175, 33.3615) -> (6.1184, 33.5605) construction
  line L739 (6.1184, 33.5605) -> (5.8729, 33.5605) construction
  spline S245 degree 3 poles (5.8729, 33.5605) (5.6275, 33.5605) (5.4285, 33.3615) (5.4285, 33.1161) knots 0 0 0 0 1 1 1 1
  line L740 (5.8729, 33.5605) -> (5.6275, 33.5605) construction
  line L741 (5.6275, 33.5605) -> (5.4285, 33.3615) construction
  line L742 (5.4285, 33.3615) -> (5.4285, 33.1161) construction
  spline S246 degree 3 poles (5.4285, 33.1161) (5.4285, 32.8706) (5.6275, 32.6715) (5.8729, 32.6715) knots 0 0 0 0 1 1 1 1
  line L743 (5.4285, 33.1161) -> (5.4285, 32.8706) construction
  line L744 (5.4285, 32.8706) -> (5.6275, 32.6715) construction
  line L745 (5.6275, 32.6715) -> (5.8729, 32.6715) construction
  spline S247 degree 3 poles (5.8729, 32.6715) (6.1184, 32.6715) (6.3175, 32.8706) (6.3175, 33.1161) knots 0 0 0 0 1 1 1 1
  line L746 (5.8729, 32.6715) -> (6.1184, 32.6715) construction
  line L747 (6.1184, 32.6715) -> (6.3175, 32.8706) construction
  line L748 (6.3175, 32.8706) -> (6.3175, 33.1161) construction
  spline S248 degree 3 poles (8.8575, 33.1161) (8.8575, 33.3615) (8.6584, 33.5605) (8.4129, 33.5605) knots 0 0 0 0 1 1 1 1
  line L749 (8.8575, 33.1161) -> (8.8575, 33.3615) construction
  line L750 (8.8575, 33.3615) -> (8.6584, 33.5605) construction
  line L751 (8.6584, 33.5605) -> (8.4129, 33.5605) construction
  spline S249 degree 3 poles (8.4129, 33.5605) (8.1675, 33.5605) (7.9685, 33.3615) (7.9685, 33.1161) knots 0 0 0 0 1 1 1 1
  line L752 (8.4129, 33.5605) -> (8.1675, 33.5605) construction
  line L753 (8.1675, 33.5605) -> (7.9685, 33.3615) construction
  line L754 (7.9685, 33.3615) -> (7.9685, 33.1161) construction
  spline S250 degree 3 poles (7.9685, 33.1161) (7.9685, 32.8706) (8.1675, 32.6715) (8.4129, 32.6715) knots 0 0 0 0 1 1 1 1
  line L755 (7.9685, 33.1161) -> (7.9685, 32.8706) construction
  line L756 (7.9685, 32.8706) -> (8.1675, 32.6715) construction
  line L757 (8.1675, 32.6715) -> (8.4129, 32.6715) construction
  spline S251 degree 3 poles (8.4129, 32.6715) (8.6584, 32.6715) (8.8575, 32.8706) (8.8575, 33.1161) knots 0 0 0 0 1 1 1 1
  line L758 (8.4129, 32.6715) -> (8.6584, 32.6715) construction
  line L759 (8.6584, 32.6715) -> (8.8575, 32.8706) construction
  line L760 (8.8575, 32.8706) -> (8.8575, 33.1161) construction
  spline S252 degree 3 poles (11.3975, 33.1161) (11.3975, 33.3615) (11.1984, 33.5605) (10.9529, 33.5605) knots 0 0 0 0 1 1 1 1
  line L761 (11.3975, 33.1161) -> (11.3975, 33.3615) construction
  line L762 (11.3975, 33.3615) -> (11.1984, 33.5605) construction
  line L763 (11.1984, 33.5605) -> (10.9529, 33.5605) construction
  spline S253 degree 3 poles (10.9529, 33.5605) (10.7075, 33.5605) (10.5085, 33.3615) (10.5085, 33.1161) knots 0 0 0 0 1 1 1 1
  line L764 (10.9529, 33.5605) -> (10.7075, 33.5605) construction
  line L765 (10.7075, 33.5605) -> (10.5085, 33.3615) construction
  line L766 (10.5085, 33.3615) -> (10.5085, 33.1161) construction
  spline S254 degree 3 poles (10.5085, 33.1161) (10.5085, 32.8706) (10.7075, 32.6715) (10.9529, 32.6715) knots 0 0 0 0 1 1 1 1
  line L767 (10.5085, 33.1161) -> (10.5085, 32.8706) construction
  line L768 (10.5085, 32.8706) -> (10.7075, 32.6715) construction
  line L769 (10.7075, 32.6715) -> (10.9529, 32.6715) construction
  spline S255 degree 3 poles (10.9529, 32.6715) (11.1984, 32.6715) (11.3975, 32.8706) (11.3975, 33.1161) knots 0 0 0 0 1 1 1 1
  line L770 (10.9529, 32.6715) -> (11.1984, 32.6715) construction
  line L771 (11.1984, 32.6715) -> (11.3975, 32.8706) construction
  line L772 (11.3975, 32.8706) -> (11.3975, 33.1161) construction
  spline S256 degree 3 poles (16.4775, 33.1161) (16.4775, 33.3615) (16.2784, 33.5605) (16.0329, 33.5605) knots 0 0 0 0 1 1 1 1
  line L773 (16.4775, 33.1161) -> (16.4775, 33.3615) construction
  line L774 (16.4775, 33.3615) -> (16.2784, 33.5605) construction
  line L775 (16.2784, 33.5605) -> (16.0329, 33.5605) construction
  spline S257 degree 3 poles (16.0329, 33.5605) (15.7875, 33.5605) (15.5885, 33.3615) (15.5885, 33.1161) knots 0 0 0 0 1 1 1 1
  line L776 (16.0329, 33.5605) -> (15.7875, 33.5605) construction
  line L777 (15.7875, 33.5605) -> (15.5885, 33.3615) construction
  line L778 (15.5885, 33.3615) -> (15.5885, 33.1161) construction
  spline S258 degree 3 poles (15.5885, 33.1161) (15.5885, 32.8706) (15.7875, 32.6715) (16.0329, 32.6715) knots 0 0 0 0 1 1 1 1
  line L779 (15.5885, 33.1161) -> (15.5885, 32.8706) construction
  line L780 (15.5885, 32.8706) -> (15.7875, 32.6715) construction
  line L781 (15.7875, 32.6715) -> (16.0329, 32.6715) construction
  spline S259 degree 3 poles (16.0329, 32.6715) (16.2784, 32.6715) (16.4775, 32.8706) (16.4775, 33.1161) knots 0 0 0 0 1 1 1 1
  line L782 (16.0329, 32.6715) -> (16.2784, 32.6715) construction
  line L783 (16.2784, 32.6715) -> (16.4775, 32.8706) construction
  line L784 (16.4775, 32.8706) -> (16.4775, 33.1161) construction
  spline S260 degree 3 poles (19.0175, 33.1161) (19.0175, 33.3615) (18.8184, 33.5605) (18.5729, 33.5605) knots 0 0 0 0 1 1 1 1
  line L785 (19.0175, 33.1161) -> (19.0175, 33.3615) construction
  line L786 (19.0175, 33.3615) -> (18.8184, 33.5605) construction
  line L787 (18.8184, 33.5605) -> (18.5729, 33.5605) construction
  spline S261 degree 3 poles (18.5729, 33.5605) (18.3275, 33.5605) (18.1285, 33.3615) (18.1285, 33.1161) knots 0 0 0 0 1 1 1 1
  line L788 (18.5729, 33.5605) -> (18.3275, 33.5605) construction
  line L789 (18.3275, 33.5605) -> (18.1285, 33.3615) construction
  line L790 (18.1285, 33.3615) -> (18.1285, 33.1161) construction
  spline S262 degree 3 poles (18.1285, 33.1161) (18.1285, 32.8706) (18.3275, 32.6715) (18.5729, 32.6715) knots 0 0 0 0 1 1 1 1
  line L791 (18.1285, 33.1161) -> (18.1285, 32.8706) construction
  line L792 (18.1285, 32.8706) -> (18.3275, 32.6715) construction
  line L793 (18.3275, 32.6715) -> (18.5729, 32.6715) construction
  spline S263 degree 3 poles (18.5729, 32.6715) (18.8184, 32.6715) (19.0175, 32.8706) (19.0175, 33.1161) knots 0 0 0 0 1 1 1 1
  line L794 (18.5729, 32.6715) -> (18.8184, 32.6715) construction
  line L795 (18.8184, 32.6715) -> (19.0175, 32.8706) construction
  line L796 (19.0175, 32.8706) -> (19.0175, 33.1161) construction
  spline S264 degree 3 poles (21.5575, 33.1161) (21.5575, 33.3615) (21.3584, 33.5605) (21.1129, 33.5605) knots 0 0 0 0 1 1 1 1
  line L797 (21.5575, 33.1161) -> (21.5575, 33.3615) construction
  line L798 (21.5575, 33.3615) -> (21.3584, 33.5605) construction
  line L799 (21.3584, 33.5605) -> (21.1129, 33.5605) construction
  spline S265 degree 3 poles (21.1129, 33.5605) (20.8675, 33.5605) (20.6685, 33.3615) (20.6685, 33.1161) knots 0 0 0 0 1 1 1 1
  line L800 (21.1129, 33.5605) -> (20.8675, 33.5605) construction
  line L801 (20.8675, 33.5605) -> (20.6685, 33.3615) construction
  line L802 (20.6685, 33.3615) -> (20.6685, 33.1161) construction
  spline S266 degree 3 poles (20.6685, 33.1161) (20.6685, 32.8706) (20.8675, 32.6715) (21.1129, 32.6715) knots 0 0 0 0 1 1 1 1
  line L803 (20.6685, 33.1161) -> (20.6685, 32.8706) construction
  line L804 (20.6685, 32.8706) -> (20.8675, 32.6715) construction
  line L805 (20.8675, 32.6715) -> (21.1129, 32.6715) construction
  spline S267 degree 3 poles (21.1129, 32.6715) (21.3584, 32.6715) (21.5575, 32.8706) (21.5575, 33.1161) knots 0 0 0 0 1 1 1 1
  line L806 (21.1129, 32.6715) -> (21.3584, 32.6715) construction
  line L807 (21.3584, 32.6715) -> (21.5575, 32.8706) construction
  line L808 (21.5575, 32.8706) -> (21.5575, 33.1161) construction
  spline S268 degree 3 poles (24.0975, 33.1161) (24.0975, 33.3615) (23.8984, 33.5605) (23.6529, 33.5605) knots 0 0 0 0 1 1 1 1
  line L809 (24.0975, 33.1161) -> (24.0975, 33.3615) construction
  line L810 (24.0975, 33.3615) -> (23.8984, 33.5605) construction
  line L811 (23.8984, 33.5605) -> (23.6529, 33.5605) construction
  spline S269 degree 3 poles (23.6529, 33.5605) (23.4075, 33.5605) (23.2085, 33.3615) (23.2085, 33.1161) knots 0 0 0 0 1 1 1 1
  line L812 (23.6529, 33.5605) -> (23.4075, 33.5605) construction
  line L813 (23.4075, 33.5605) -> (23.2085, 33.3615) construction
  line L814 (23.2085, 33.3615) -> (23.2085, 33.1161) construction
  spline S270 degree 3 poles (23.2085, 33.1161) (23.2085, 32.8706) (23.4075, 32.6715) (23.6529, 32.6715) knots 0 0 0 0 1 1 1 1
  line L815 (23.2085, 33.1161) -> (23.2085, 32.8706) construction
  line L816 (23.2085, 32.8706) -> (23.4075, 32.6715) construction
  line L817 (23.4075, 32.6715) -> (23.6529, 32.6715) construction
  spline S271 degree 3 poles (23.6529, 32.6715) (23.8984, 32.6715) (24.0975, 32.8706) (24.0975, 33.1161) knots 0 0 0 0 1 1 1 1
  line L818 (23.6529, 32.6715) -> (23.8984, 32.6715) construction
  line L819 (23.8984, 32.6715) -> (24.0975, 32.8706) construction
  line L820 (24.0975, 32.8706) -> (24.0975, 33.1161) construction
  spline S272 degree 3 poles (13.9375, 33.1161) (13.9375, 33.3615) (13.7384, 33.5605) (13.4929, 33.5605) knots 0 0 0 0 1 1 1 1
  line L821 (13.9375, 33.1161) -> (13.9375, 33.3615) construction
  line L822 (13.9375, 33.3615) -> (13.7384, 33.5605) construction
  line L823 (13.7384, 33.5605) -> (13.4929, 33.5605) construction
  spline S273 degree 3 poles (13.4929, 33.5605) (13.2475, 33.5605) (13.0485, 33.3615) (13.0485, 33.1161) knots 0 0 0 0 1 1 1 1
  line L824 (13.4929, 33.5605) -> (13.2475, 33.5605) construction
  line L825 (13.2475, 33.5605) -> (13.0485, 33.3615) construction
  line L826 (13.0485, 33.3615) -> (13.0485, 33.1161) construction
  spline S274 degree 3 poles (13.0485, 33.1161) (13.0485, 32.8706) (13.2475, 32.6715) (13.4929, 32.6715) knots 0 0 0 0 1 1 1 1
  line L827 (13.0485, 33.1161) -> (13.0485, 32.8706) construction
  line L828 (13.0485, 32.8706) -> (13.2475, 32.6715) construction
  line L829 (13.2475, 32.6715) -> (13.4929, 32.6715) construction
  spline S275 degree 3 poles (13.4929, 32.6715) (13.7384, 32.6715) (13.9375, 32.8706) (13.9375, 33.1161) knots 0 0 0 0 1 1 1 1
  line L830 (13.4929, 32.6715) -> (13.7384, 32.6715) construction
  line L831 (13.7384, 32.6715) -> (13.9375, 32.8706) construction
  line L832 (13.9375, 32.8706) -> (13.9375, 33.1161) construction
  spline S276 degree 3 poles (3.7139, 24.2261) (3.7139, 24.8572) (3.2021, 25.369) (2.571, 25.369) knots 0 0 0 0 1 1 1 1
  line L833 (3.7139, 24.2261) -> (3.7139, 24.8572) construction
  line L834 (3.7139, 24.8572) -> (3.2021, 25.369) construction
  line L835 (3.2021, 25.369) -> (2.571, 25.369) construction
  spline S277 degree 3 poles (2.571, 25.369) (1.9399, 25.369) (1.4279, 24.8572) (1.4279, 24.2261) knots 0 0 0 0 1 1 1 1
  line L836 (2.571, 25.369) -> (1.9399, 25.369) construction
  line L837 (1.9399, 25.369) -> (1.4279, 24.8572) construction
  line L838 (1.4279, 24.8572) -> (1.4279, 24.2261) construction
  spline S278 degree 3 poles (1.4279, 24.2261) (1.4279, 23.5949) (1.9399, 23.083) (2.571, 23.083) knots 0 0 0 0 1 1 1 1
  line L839 (1.4279, 24.2261) -> (1.4279, 23.5949) construction
  line L840 (1.4279, 23.5949) -> (1.9399, 23.083) construction
  line L841 (1.9399, 23.083) -> (2.571, 23.083) construction
  spline S279 degree 3 poles (2.571, 23.083) (3.2021, 23.083) (3.7139, 23.5949) (3.7139, 24.2261) knots 0 0 0 0 1 1 1 1
  line L842 (2.571, 23.083) -> (3.2021, 23.083) construction
  line L843 (3.2021, 23.083) -> (3.7139, 23.5949) construction
  line L844 (3.7139, 23.5949) -> (3.7139, 24.2261) construction
  spline S280 degree 3 poles (28.0979, 24.2261) (28.0979, 24.8572) (27.5861, 25.369) (26.955, 25.369) knots 0 0 0 0 1 1 1 1
  line L845 (28.0979, 24.2261) -> (28.0979, 24.8572) construction
  line L846 (28.0979, 24.8572) -> (27.5861, 25.369) construction
  line L847 (27.5861, 25.369) -> (26.955, 25.369) construction
  spline S281 degree 3 poles (26.955, 25.369) (26.3239, 25.369) (25.812, 24.8572) (25.812, 24.2261) knots 0 0 0 0 1 1 1 1
  line L848 (26.955, 25.369) -> (26.3239, 25.369) construction
  line L849 (26.3239, 25.369) -> (25.812, 24.8572) construction
  line L850 (25.812, 24.8572) -> (25.812, 24.2261) construction
  spline S282 degree 3 poles (25.812, 24.2261) (25.812, 23.5949) (26.3239, 23.083) (26.955, 23.083) knots 0 0 0 0 1 1 1 1
  line L851 (25.812, 24.2261) -> (25.812, 23.5949) construction
  line L852 (25.812, 23.5949) -> (26.3239, 23.083) construction
  line L853 (26.3239, 23.083) -> (26.955, 23.083) construction
  spline S283 degree 3 poles (26.955, 23.083) (27.5861, 23.083) (28.0979, 23.5949) (28.0979, 24.2261) knots 0 0 0 0 1 1 1 1
  line L854 (26.955, 23.083) -> (27.5861, 23.083) construction
  line L855 (27.5861, 23.083) -> (28.0979, 23.5949) construction
  line L856 (28.0979, 23.5949) -> (28.0979, 24.2261) construction
  line L857 (8.4129, 32.735) -> (8.4129, 33.1161)
  line L858 (2.571, 25.369) -> (2.571, 23.0323)
  line L859 (1.4279, 24.2261) -> (3.7139, 24.2261)
  circle A0 centre (2.5709, 24.2261) radius 1.1429
  line L860 (26.955, 25.369) -> (26.955, 23.083)
  line L861 (25.812, 24.2261) -> (28.0979, 24.2261)
  circle A1 centre (26.955, 24.2261) radius 1.1429
  point P0 (0, 0)
  dimension "d1" = 21.59
  constraints: 20 end point, 3 perpendicular, 2 midpoint, 1 parallel, 858 other
  measures "d1" distance of L15.start L15.end
sketch "Sketch2" plane through (0, 0, 0) normal (0, 1, 0) x (-1, 0, 0)
  line L0 (10.795, 10.4409) -> (-10.795, 10.4409)
  line L1 (-14.351, 6.8848) -> (-14.351, -6.8848)
  line L2 (-10.5408, -10.3871) -> (10.7952, -10.3871)
  line L3 (14.6273, 7.2608) -> (14.6273, -6.6157)
  circle A0 centre (-12.0651, 0.0269) radius 1.1429
  circle A1 centre (12.319, 0.0269) radius 1.1429
  arc A2 (-10.795, 10.4409) -> (-14.351, 6.8848) centre (-10.795, 6.8848) ccw
  arc A3 (14.6273, 7.2608) -> (10.795, 10.4409) centre (11.3918, 7.2608) ccw
  arc A4 (10.7952, -10.3871) -> (14.6273, -6.6157) centre (10.8554, -6.6157) ccw
  arc A5 (-14.351, -6.8848) -> (-10.5408, -10.3871) centre (-10.8363, -6.8848) ccw
  line L4 (-14.351, 0) -> (14.6273, 0) construction
  line L5 (0, 10.4409) -> (0, -10.3871) construction
  line L6 (-10.795, 10.9409) -> (10.7502, 10.9409)
  arc A6 (15.1273, 7.2608) -> (10.7502, 10.9409) centre (11.3918, 7.2608) ccw
  line L7 (15.1273, 7.2608) -> (15.1273, -6.6157)
  arc A7 (10.7913, -10.8871) -> (15.1273, -6.6157) centre (10.8554, -6.6157) ccw
  line L8 (10.7913, -10.8871) -> (-10.5205, -10.8871)
  arc A8 (-14.851, -6.8848) -> (-10.5205, -10.8871) centre (-10.8363, -6.8848) ccw
  line L9 (-14.851, -6.8848) -> (-14.851, 6.8848)
  arc A9 (-10.795, 10.9409) -> (-14.851, 6.8848) centre (-10.795, 6.8848) ccw
  line L10 (10.5957, 12.9409) -> (-10.795, 12.9409)
  arc A10 (-10.795, 12.9409) -> (-16.851, 6.8848) centre (-10.795, 6.8848) ccw
  line L11 (-16.851, 6.8848) -> (-16.851, -6.8848)
  arc A11 (-16.851, -6.8848) -> (-10.4496, -12.8871) centre (-10.8363, -6.8848) ccw
  line L12 (-10.4496, -12.8871) -> (10.7778, -12.8871)
  arc A12 (10.7778, -12.8871) -> (17.1273, -6.6157) centre (10.8554, -6.6157) ccw
  line L13 (17.1273, -6.6157) -> (17.1273, 7.2608)
  arc A13 (17.1273, 7.2608) -> (10.5957, 12.9409) centre (11.3918, 7.2608) ccw
  circle A14 centre (-12.0651, 0.0269) radius 1.7429
  arc A15 (-14.851, -2.4727) -> (-14.851, 2.5265) centre (-12.0651, 0.0269) ccw
  circle A16 centre (12.319, 0.0269) radius 1.7429
  arc A17 (15.1273, 2.5013) -> (15.1273, -2.4475) centre (12.319, 0.0269) ccw
  arc A18 (-14.851, 2.5265) -> (-14.851, -2.4727) centre (-12.0651, 0.0269) ccw
  arc A19 (15.1273, -2.4475) -> (15.1273, 2.5013) centre (12.319, 0.0269) ccw
  line L14 (-10.3221, 15.9323) -> (-10.3221, -15.3986)
  line L15 (10.5761, 15.9323) -> (10.5761, -15.3986)
  point P0 (0, 0)
  point P1 (0, 0)
  dimension "d2" = 0.5
  dimension "d3" = 2
  dimension "d4" = 0.6
  dimension "d5" = 2
  dimension "d6" = 0.6
  dimension "d8" = 2
  constraints: 32 end point, 32 point on circle, 20 centre point, 8 point on line, 5 tangent, 3 horizontal, 3 vertical, 2 midpoint, 2 parallel, 2 perpendicular, 40 other
  measures "d2" distance between parallel lines of L0 L6
  measures "d3" distance between parallel lines of L6 L10
  measures "d4" radial gap between concentric circles of A14 A0
  measures "d5" radial gap between concentric circles of A14 A15
  measures "d6" radial gap between concentric circles of A1 A16
  measures "d8" radial gap between concentric circles of A16 A17
extrude "Extrusion1" add sketch "Sketch2" along normal blind 1.5 contours A3 L3 A17 L15 L0 | L0 L15 L6 A6 L7 A17 L3 A3 | L15 A17 L2 L14 A15 L0 | L0 L14 L6 L15 | L14 A15 L1 A2 L0 | L0 A2 L1 A15 L9 A9 L6 L14 | L15 L10 A13 L13 A12 L12 L8 A7 L7 A19 A6 L6 | L6 L14 L10 L15 | L15 A17 | A16 | A17 L3 L15 | A17 L7 L3 | L6 A9 L9 A18 A8 L8 L14 L12 A11 L11 A10 L10 | A14 | L14 A15 L1 | A15 L14 | A17 L3 A4 L2 L15 | A17 L7 A7 L8 L15 L2 A4 L3 | A19 L7 | L14 L2 A5 L1 A15 | L1 A15 L9 | L15 L8 L14 L2 | L1 A5 L2 L14 L8 A8 L9 A15 | L9 A18 | L15 L12 L14 L8 | A0 | A1
extrude "Extrusion2" cut sketch "Sketch2" along normal blind 1.5 contours A16 | A14 | A0 | A1
extrude "Extrusion3" add sketch "Sketch2" along normal blind 3 contours L15 A17 | A17 L3 L15 | A17 L7 L3 | L14 A15 L1 | A15 L14 | A19 L7 | L1 A15 L9 | L9 A18
extrude "Extrusion4" add sketch "Sketch2" along normal blind 5 contours L15 L10 A13 L13 A12 L12 L8 A7 L7 A19 A6 L6 | L6 L14 L10 L15 | L6 A9 L9 A18 A8 L8 L14 L12 A11 L11 A10 L10 | A19 L7 | L9 A18 | L15 L12 L14 L8
ref_plane "Work Plane1" through (0, 1.5, 0) normal (0, 1, 0) x (-1, 0, 0)
sketch "Sketch3" plane through (0, 1.5, 0) normal (0, 1, 0) x (-1, 0, 0)
  line L0 (-10.3221, 15.9323) -> (-10.3221, -15.3986) projected
  line L1 (10.5761, 15.9323) -> (10.5761, -15.3986) projected
  line L2 (-10.3221, 14.4484) -> (10.5761, 14.4484)
  line L3 (10.5761, 14.4484) -> (10.5761, 8.2696)
  line L4 (10.5761, 8.2696) -> (-10.3221, 8.2696)
  line L5 (-10.3221, 8.2696) -> (-10.3221, 14.4484)
  line L6 (-10.3221, -8.2072) -> (10.5761, -8.2072)
  line L7 (10.5761, -8.2072) -> (10.5761, -14.3236)
  line L8 (10.5761, -14.3236) -> (-10.3221, -14.3236)
  line L9 (-10.3221, -14.3236) -> (-10.3221, -8.2072)
  point P0 (0, 0)
  constraints: 16 end point, 4 parallel, 4 point on line, 2 horizontal, 2 perpendicular
extrude "Extrusion5" cut sketch "Sketch3" along normal blind 5 contours L2 L1 L4 L0 | L6 L1 L8 L0
fillet "Fillet1" radius 2 4 edges at (-10.5761, 5, 11.9409) (-10.5761, 5, -11.8871) (10.3221, 5, -11.8871) (10.3221, 5, 11.9409)